Autodesk Fusion 360 part; units mm, degrees
note: some values were not read from the file. Chosen so that the rebuilt part matches the saved one: which face or edge a step refers to. Set by a fixed rule: which sketch regions a step uses.
(part 2 of 4)
sketch "Front projection" plane through (0, 0, 0) normal (0, 0, 1) x (1, 0, 0) in component "Front"
  arc A0 (5.175, 6.81) -> (5.175, 8.2242) centre (4.4679, 7.5171) ccw
  line L0 (5.175, 6.81) -> (5.175, 5.175)
  line L1 (5.175, 58.825) -> (5.175, 57.19)
  arc A1 (5.175, 55.7758) -> (5.175, 57.19) centre (4.4679, 56.4829) ccw
  line L2 (5.175, 55.7758) -> (5.175, 48.2242)
  arc A2 (3.5613, 47.095) -> (5.175, 48.2242) centre (4.4679, 47.5171) ccw
  line L3 (3.5613, 47.095) -> (2, 47.095)
  line L4 (2, 36.905) -> (3.5613, 36.905)
  arc A3 (5.175, 35.7758) -> (3.5613, 36.905) centre (4.4679, 36.4829) ccw
  line L5 (5.175, 35.7758) -> (5.175, 28.2242)
  arc A4 (3.5613, 27.095) -> (5.175, 28.2242) centre (4.4679, 27.5171) ccw
  line L6 (3.5613, 27.095) -> (2, 27.095)
  line L7 (2, 16.905) -> (3.5613, 16.905)
  arc A5 (5.175, 15.7758) -> (3.5613, 16.905) centre (4.4679, 16.4829) ccw
  line L8 (5.175, 15.7758) -> (5.175, 8.2242)
  line L9 (15.7758, 58.825) -> (5.175, 58.825)
  line L10 (2, 16.905) -> (2, 27.095)
  arc A6 (238.825, 8.2242) -> (238.825, 6.81) centre (239.5321, 7.5171) ccw
  line L11 (216.905, 62) -> (216.905, 60.4387)
  arc A7 (215.7758, 58.825) -> (216.905, 60.4387) centre (216.4829, 59.5321) ccw
  line L12 (215.7758, 58.825) -> (208.2242, 58.825)
  arc A8 (207.095, 60.4387) -> (208.2242, 58.825) centre (207.5171, 59.5321) ccw
  line L13 (207.095, 60.4387) -> (207.095, 62)
  line L14 (196.905, 62) -> (196.905, 60.4387)
  arc A9 (195.7758, 58.825) -> (196.905, 60.4387) centre (196.4829, 59.5321) ccw
  line L15 (195.7758, 58.825) -> (188.2242, 58.825)
  arc A10 (187.095, 60.4387) -> (188.2242, 58.825) centre (187.5171, 59.5321) ccw
  line L16 (187.095, 60.4387) -> (187.095, 62)
  line L17 (176.905, 62) -> (176.905, 60.4387)
  arc A11 (175.7758, 58.825) -> (176.905, 60.4387) centre (176.4829, 59.5321) ccw
  line L18 (175.7758, 58.825) -> (168.2242, 58.825)
  arc A12 (167.095, 60.4387) -> (168.2242, 58.825) centre (167.5171, 59.5321) ccw
  line L19 (167.095, 60.4387) -> (167.095, 62)
  line L20 (156.905, 62) -> (156.905, 60.4387)
  arc A13 (155.7758, 58.825) -> (156.905, 60.4387) centre (156.4829, 59.5321) ccw
  line L21 (155.7758, 58.825) -> (148.2242, 58.825)
  arc A14 (147.095, 60.4387) -> (148.2242, 58.825) centre (147.5171, 59.5321) ccw
  line L22 (147.095, 60.4387) -> (147.095, 62)
  line L23 (136.905, 62) -> (136.905, 60.4387)
  arc A15 (135.7758, 58.825) -> (136.905, 60.4387) centre (136.4829, 59.5321) ccw
  line L24 (135.7758, 58.825) -> (128.2242, 58.825)
  arc A16 (127.095, 60.4387) -> (128.2242, 58.825) centre (127.5171, 59.5321) ccw
  line L25 (127.095, 60.4387) -> (127.095, 62)
  line L26 (116.905, 62) -> (116.905, 60.4387)
  arc A17 (115.7758, 58.825) -> (116.905, 60.4387) centre (116.4829, 59.5321) ccw
  line L27 (115.7758, 58.825) -> (108.2242, 58.825)
  arc A18 (107.095, 60.4387) -> (108.2242, 58.825) centre (107.5171, 59.5321) ccw
  line L28 (107.095, 60.4387) -> (107.095, 62)
  line L29 (96.905, 62) -> (96.905, 60.4387)
  arc A19 (95.7758, 58.825) -> (96.905, 60.4387) centre (96.4829, 59.5321) ccw
  line L30 (95.7758, 58.825) -> (88.2242, 58.825)
  arc A20 (87.095, 60.4387) -> (88.2242, 58.825) centre (87.5171, 59.5321) ccw
  line L31 (87.095, 60.4387) -> (87.095, 62)
  line L32 (76.905, 62) -> (76.905, 60.4387)
  arc A21 (75.7758, 58.825) -> (76.905, 60.4387) centre (76.4829, 59.5321) ccw
  line L33 (75.7758, 58.825) -> (68.2242, 58.825)
  arc A22 (67.095, 60.4387) -> (68.2242, 58.825) centre (67.5171, 59.5321) ccw
  line L34 (67.095, 60.4387) -> (67.095, 62)
  line L35 (56.905, 62) -> (56.905, 60.4387)
  arc A23 (55.7758, 58.825) -> (56.905, 60.4387) centre (56.4829, 59.5321) ccw
  line L36 (55.7758, 58.825) -> (48.2242, 58.825)
  arc A24 (47.095, 60.4387) -> (48.2242, 58.825) centre (47.5171, 59.5321) ccw
  line L37 (47.095, 60.4387) -> (47.095, 62)
  line L38 (238.825, 58.825) -> (228.2242, 58.825)
  arc A25 (227.095, 60.4387) -> (228.2242, 58.825) centre (227.5171, 59.5321) ccw
  line L39 (227.095, 60.4387) -> (227.095, 62)
  line L40 (36.905, 62) -> (36.905, 60.4387)
  arc A26 (35.7758, 58.825) -> (36.905, 60.4387) centre (36.4829, 59.5321) ccw
  line L41 (35.7758, 58.825) -> (28.2242, 58.825)
  arc A27 (27.095, 60.4387) -> (28.2242, 58.825) centre (27.5171, 59.5321) ccw
  line L42 (27.095, 60.4387) -> (27.095, 62)
  line L43 (16.905, 62) -> (16.905, 60.4387)
  arc A28 (15.7758, 58.825) -> (16.905, 60.4387) centre (16.4829, 59.5321) ccw
  line L44 (238.825, 5.175) -> (238.825, 6.81)
  line L45 (238.825, 58.825) -> (238.825, 57.19)
  line L46 (16.905, 62) -> (27.095, 62)
  line L47 (36.905, 62) -> (47.095, 62)
  line L48 (56.905, 62) -> (67.095, 62)
  line L49 (76.905, 62) -> (87.095, 62)
  line L50 (96.905, 62) -> (107.095, 62)
  line L51 (116.905, 62) -> (127.095, 62)
  line L52 (136.905, 62) -> (147.095, 62)
  line L53 (156.905, 62) -> (167.095, 62)
  line L54 (176.905, 62) -> (187.095, 62)
  line L55 (196.905, 62) -> (207.095, 62)
  line L56 (216.905, 62) -> (227.095, 62)
  arc A29 (238.825, 57.19) -> (238.825, 55.7758) centre (239.5321, 56.4829) ccw
  line L57 (238.825, 55.7758) -> (238.825, 48.2242)
  arc A30 (238.825, 48.2242) -> (240.4387, 47.095) centre (239.5321, 47.5171) ccw
  line L58 (240.4387, 47.095) -> (242, 47.095)
  line L59 (242, 47.095) -> (242, 36.905)
  line L60 (240.4387, 36.905) -> (242, 36.905)
  arc A31 (240.4387, 36.905) -> (238.825, 35.7758) centre (239.5321, 36.4829) ccw
  line L61 (238.825, 28.2242) -> (238.825, 35.7758)
  arc A32 (238.825, 28.2242) -> (240.4387, 27.095) centre (239.5321, 27.5171) ccw
  line L62 (242, 27.095) -> (240.4387, 27.095)
  line L63 (242, 27.095) -> (242, 16.905)
  line L64 (240.4387, 16.905) -> (242, 16.905)
  arc A33 (240.4387, 16.905) -> (238.825, 15.7758) centre (239.5321, 16.4829) ccw
  line L65 (238.825, 8.2242) -> (238.825, 15.7758)
  line L66 (238.825, 5.175) -> (228.2242, 5.175)
  arc A34 (228.2242, 5.175) -> (227.095, 3.5613) centre (227.5171, 4.4679) ccw
  line L67 (227.095, 3.5613) -> (227.095, 2)
  line L68 (227.095, 2) -> (216.905, 2)
  line L69 (216.905, 3.5613) -> (216.905, 2)
  arc A35 (216.905, 3.5613) -> (215.7758, 5.175) centre (216.4829, 4.4679) ccw
  line L70 (208.2242, 5.175) -> (215.7758, 5.175)
  arc A36 (208.2242, 5.175) -> (207.095, 3.5613) centre (207.5171, 4.4679) ccw
  line L71 (207.095, 2) -> (207.095, 3.5613)
  line L72 (207.095, 2) -> (196.905, 2)
  line L73 (196.905, 3.5613) -> (196.905, 2)
  arc A37 (196.905, 3.5613) -> (195.7758, 5.175) centre (196.4829, 4.4679) ccw
  line L74 (188.2242, 5.175) -> (195.7758, 5.175)
  arc A38 (188.2242, 5.175) -> (187.095, 3.5613) centre (187.5171, 4.4679) ccw
  line L75 (187.095, 2) -> (187.095, 3.5613)
  line L76 (187.095, 2) -> (176.905, 2)
  line L77 (176.905, 3.5613) -> (176.905, 2)
  arc A39 (176.905, 3.5613) -> (175.7758, 5.175) centre (176.4829, 4.4679) ccw
  line L78 (168.2242, 5.175) -> (175.7758, 5.175)
  arc A40 (168.2242, 5.175) -> (167.095, 3.5613) centre (167.5171, 4.4679) ccw
  line L79 (167.095, 2) -> (167.095, 3.5613)
  line L80 (167.095, 2) -> (156.905, 2)
  line L81 (156.905, 3.5613) -> (156.905, 2)
  arc A41 (156.905, 3.5613) -> (155.7758, 5.175) centre (156.4829, 4.4679) ccw
  line L82 (148.2242, 5.175) -> (155.7758, 5.175)
  arc A42 (148.2242, 5.175) -> (147.095, 3.5613) centre (147.5171, 4.4679) ccw
  line L83 (147.095, 2) -> (147.095, 3.5613)
  line L84 (147.095, 2) -> (136.905, 2)
  line L85 (136.905, 3.5613) -> (136.905, 2)
  arc A43 (136.905, 3.5613) -> (135.7758, 5.175) centre (136.4829, 4.4679) ccw
  line L86 (128.2242, 5.175) -> (135.7758, 5.175)
  arc A44 (128.2242, 5.175) -> (127.095, 3.5613) centre (127.5171, 4.4679) ccw
  line L87 (127.095, 2) -> (127.095, 3.5613)
  line L88 (127.095, 2) -> (116.905, 2)
  line L89 (116.905, 3.5613) -> (116.905, 2)
  arc A45 (116.905, 3.5613) -> (115.7758, 5.175) centre (116.4829, 4.4679) ccw
  line L90 (108.2242, 5.175) -> (115.7758, 5.175)
  arc A46 (108.2242, 5.175) -> (107.095, 3.5613) centre (107.5171, 4.4679) ccw
  line L91 (107.095, 2) -> (107.095, 3.5613)
  line L92 (107.095, 2) -> (96.905, 2)
  line L93 (96.905, 3.5613) -> (96.905, 2)
  arc A47 (96.905, 3.5613) -> (95.7758, 5.175) centre (96.4829, 4.4679) ccw
  line L94 (88.2242, 5.175) -> (95.7758, 5.175)
  arc A48 (88.2242, 5.175) -> (87.095, 3.5613) centre (87.5171, 4.4679) ccw
  line L95 (87.095, 2) -> (87.095, 3.5613)
  line L96 (87.095, 2) -> (76.905, 2)
  line L97 (76.905, 3.5613) -> (76.905, 2)
  arc A49 (76.905, 3.5613) -> (75.7758, 5.175) centre (76.4829, 4.4679) ccw
  line L98 (68.2242, 5.175) -> (75.7758, 5.175)
  arc A50 (68.2242, 5.175) -> (67.095, 3.5613) centre (67.5171, 4.4679) ccw
  line L99 (67.095, 2) -> (67.095, 3.5613)
  line L100 (67.095, 2) -> (56.905, 2)
  line L101 (56.905, 3.5613) -> (56.905, 2)
  arc A51 (56.905, 3.5613) -> (55.7758, 5.175) centre (56.4829, 4.4679) ccw
  line L102 (48.2242, 5.175) -> (55.7758, 5.175)
  arc A52 (48.2242, 5.175) -> (47.095, 3.5613) centre (47.5171, 4.4679) ccw
  line L103 (47.095, 2) -> (47.095, 3.5613)
  line L104 (47.095, 2) -> (36.905, 2)
  line L105 (36.905, 3.5613) -> (36.905, 2)
  arc A53 (36.905, 3.5613) -> (35.7758, 5.175) centre (36.4829, 4.4679) ccw
  line L106 (28.2242, 5.175) -> (35.7758, 5.175)
  arc A54 (28.2242, 5.175) -> (27.095, 3.5613) centre (27.5171, 4.4679) ccw
  line L107 (27.095, 2) -> (27.095, 3.5613)
  line L108 (27.095, 2) -> (16.905, 2)
  line L109 (16.905, 3.5613) -> (16.905, 2)
  arc A55 (16.905, 3.5613) -> (15.7758, 5.175) centre (16.4829, 4.4679) ccw
  line L110 (5.175, 5.175) -> (15.7758, 5.175)
  line L111 (2, 36.905) -> (2, 47.095)
sketch "Right Projection" plane through (0, 0, 0) normal (0, 0, 1) x (1, 0, 0) in component "Right"
  line L0 (-300.4387, 26.095) -> (-302, 26.095)
  line L1 (-302, 35.905) -> (-300.4387, 35.905)
  arc A0 (-298.825, 34.7758) -> (-300.4387, 35.905) centre (-299.5321, 35.4829) ccw
  line L2 (-298.825, 34.7758) -> (-298.825, 27.2242)
  arc A1 (-300.4387, 26.095) -> (-298.825, 27.2242) centre (-299.5321, 26.5171) ccw
  line L3 (-302, 55.905) -> (-300.4387, 55.905)
  line L4 (-300.4387, 46.095) -> (-302, 46.095)
  arc A2 (-300.4387, 46.095) -> (-298.825, 47.2242) centre (-299.5321, 46.5171) ccw
  line L5 (-298.825, 54.7758) -> (-298.825, 47.2242)
  arc A3 (-298.825, 54.7758) -> (-300.4387, 55.905) centre (-299.5321, 55.4829) ccw
  line L6 (-302, 75.905) -> (-300.4387, 75.905)
  line L7 (-300.4387, 66.095) -> (-302, 66.095)
  arc A4 (-300.4387, 66.095) -> (-298.825, 67.2242) centre (-299.5321, 66.5171) ccw
  line L8 (-298.825, 74.7758) -> (-298.825, 67.2242)
  arc A5 (-298.825, 74.7758) -> (-300.4387, 75.905) centre (-299.5321, 75.4829) ccw
  line L9 (-302, 95.905) -> (-300.4387, 95.905)
  line L10 (-300.4387, 86.095) -> (-302, 86.095)
  arc A6 (-300.4387, 86.095) -> (-298.825, 87.2242) centre (-299.5321, 86.5171) ccw
  line L11 (-298.825, 94.7758) -> (-298.825, 87.2242)
  arc A7 (-298.825, 94.7758) -> (-300.4387, 95.905) centre (-299.5321, 95.4829) ccw
  line L12 (-302, 115.905) -> (-300.4387, 115.905)
  line L13 (-300.4387, 106.095) -> (-302, 106.095)
  arc A8 (-300.4387, 106.095) -> (-298.825, 107.2242) centre (-299.5321, 106.5171) ccw
  line L14 (-298.825, 114.7758) -> (-298.825, 107.2242)
  arc A9 (-298.825, 114.7758) -> (-300.4387, 115.905) centre (-299.5321, 115.4829) ccw
  line L15 (-302, 135.905) -> (-300.4387, 135.905)
  line L16 (-300.4387, 126.095) -> (-302, 126.095)
  arc A10 (-300.4387, 126.095) -> (-298.825, 127.2242) centre (-299.5321, 126.5171) ccw
  line L17 (-298.825, 134.7758) -> (-298.825, 127.2242)
  arc A11 (-298.825, 134.7758) -> (-300.4387, 135.905) centre (-299.5321, 135.4829) ccw
  line L18 (-302, 155.905) -> (-300.4387, 155.905)
  line L19 (-300.4387, 166.095) -> (-302, 166.095)
  arc A12 (-300.4387, 166.095) -> (-298.825, 167.2242) centre (-299.5321, 166.5171) ccw
  line L20 (-298.825, 182) -> (-298.825, 167.2242)
  line L21 (-298.825, 14.7758) -> (-298.825, 0)
  arc A13 (-298.825, 14.7758) -> (-300.4387, 15.905) centre (-299.5321, 15.4829) ccw
  line L22 (-302, 15.905) -> (-300.4387, 15.905)
  line L23 (-300.4387, 146.095) -> (-302, 146.095)
  arc A14 (-300.4387, 146.095) -> (-298.825, 147.2242) centre (-299.5321, 146.5171) ccw
  line L24 (-298.825, 154.7758) -> (-298.825, 147.2242)
  arc A15 (-298.825, 154.7758) -> (-300.4387, 155.905) centre (-299.5321, 155.4829) ccw
  line L25 (-298.825, 0) -> (-286.905, 0)
  line L26 (-302, 26.095) -> (-302, 15.905)
  line L27 (-302, 46.095) -> (-302, 35.905)
  line L28 (-302, 66.095) -> (-302, 55.905)
  line L29 (-302, 86.095) -> (-302, 75.905)
  line L30 (-302, 106.095) -> (-302, 95.905)
  line L31 (-302, 126.095) -> (-302, 115.905)
  line L32 (-302, 146.095) -> (-302, 135.905)
  line L33 (-302, 166.095) -> (-302, 155.905)
  line L34 (-286.905, 182) -> (-298.825, 182)
  line L35 (-286.905, 182) -> (-286.905, 180.4387)
  arc A16 (-286.905, 180.4387) -> (-285.7758, 178.825) centre (-286.4829, 179.5321) ccw
  line L36 (-285.7758, 178.825) -> (-278.2242, 178.825)
  arc A17 (-278.2242, 178.825) -> (-277.095, 180.4387) centre (-277.5171, 179.5321) ccw
  line L37 (-277.095, 180.4387) -> (-277.095, 182)
  line L38 (-266.905, 182) -> (-277.095, 182)
  line L39 (-266.905, 182) -> (-266.905, 180.4387)
  arc A18 (-266.905, 180.4387) -> (-265.7758, 178.825) centre (-266.4829, 179.5321) ccw
  line L40 (-265.7758, 178.825) -> (-258.2242, 178.825)
  arc A19 (-258.2242, 178.825) -> (-257.095, 180.4387) centre (-257.5171, 179.5321) ccw
  line L41 (-257.095, 180.4387) -> (-257.095, 182)
  line L42 (-245.175, 182) -> (-257.095, 182)
  line L43 (-245.175, 182) -> (-245.175, 167.2242)
  arc A20 (-245.175, 167.2242) -> (-243.5613, 166.095) centre (-244.4679, 166.5171) ccw
  line L44 (-243.5613, 166.095) -> (-242, 166.095)
  line L45 (-242, 155.905) -> (-242, 166.095)
  line L46 (-242, 155.905) -> (-243.5613, 155.905)
  arc A21 (-243.5613, 155.905) -> (-245.175, 154.7758) centre (-244.4679, 155.4829) ccw
  line L47 (-245.175, 154.7758) -> (-245.175, 147.2242)
  arc A22 (-245.175, 147.2242) -> (-243.5613, 146.095) centre (-244.4679, 146.5171) ccw
  line L48 (-243.5613, 146.095) -> (-242, 146.095)
  line L49 (-242, 135.905) -> (-242, 146.095)
  line L50 (-242, 135.905) -> (-243.5613, 135.905)
  arc A23 (-243.5613, 135.905) -> (-245.175, 134.7758) centre (-244.4679, 135.4829) ccw
  line L51 (-245.175, 134.7758) -> (-245.175, 127.2242)
  arc A24 (-245.175, 127.2242) -> (-243.5613, 126.095) centre (-244.4679, 126.5171) ccw
  line L52 (-243.5613, 126.095) -> (-242, 126.095)
  line L53 (-242, 115.905) -> (-242, 126.095)
  line L54 (-242, 115.905) -> (-243.5613, 115.905)
  arc A25 (-243.5613, 115.905) -> (-245.175, 114.7758) centre (-244.4679, 115.4829) ccw
  line L55 (-245.175, 114.7758) -> (-245.175, 107.2242)
  arc A26 (-245.175, 107.2242) -> (-243.5613, 106.095) centre (-244.4679, 106.5171) ccw
  line L56 (-243.5613, 106.095) -> (-242, 106.095)
  line L57 (-242, 95.905) -> (-242, 106.095)
  line L58 (-242, 95.905) -> (-243.5613, 95.905)
  arc A27 (-243.5613, 95.905) -> (-245.175, 94.7758) centre (-244.4679, 95.4829) ccw
  line L59 (-245.175, 94.7758) -> (-245.175, 87.2242)
  arc A28 (-245.175, 87.2242) -> (-243.5613, 86.095) centre (-244.4679, 86.5171) ccw
  line L60 (-243.5613, 86.095) -> (-242, 86.095)
  line L61 (-242, 75.905) -> (-242, 86.095)
  line L62 (-242, 75.905) -> (-243.5613, 75.905)
  arc A29 (-243.5613, 75.905) -> (-245.175, 74.7758) centre (-244.4679, 75.4829) ccw
  line L63 (-245.175, 74.7758) -> (-245.175, 67.2242)
  arc A30 (-245.175, 67.2242) -> (-243.5613, 66.095) centre (-244.4679, 66.5171) ccw
  line L64 (-243.5613, 66.095) -> (-242, 66.095)
  line L65 (-242, 55.905) -> (-242, 66.095)
  line L66 (-242, 55.905) -> (-243.5613, 55.905)
  arc A31 (-243.5613, 55.905) -> (-245.175, 54.7758) centre (-244.4679, 55.4829) ccw
  line L67 (-245.175, 54.7758) -> (-245.175, 47.2242)
  arc A32 (-245.175, 47.2242) -> (-243.5613, 46.095) centre (-244.4679, 46.5171) ccw
  line L68 (-243.5613, 46.095) -> (-242, 46.095)
  line L69 (-242, 35.905) -> (-242, 46.095)
  line L70 (-243.5613, 35.905) -> (-242, 35.905)
  arc A33 (-243.5613, 35.905) -> (-245.175, 34.7758) centre (-244.4679, 35.4829) ccw
  line L71 (-245.175, 27.2242) -> (-245.175, 34.7758)
  arc A34 (-245.175, 27.2242) -> (-243.5613, 26.095) centre (-244.4679, 26.5171) ccw
  line L72 (-242, 26.095) -> (-243.5613, 26.095)
  line L73 (-242, 15.905) -> (-242, 26.095)
  line L74 (-243.5613, 15.905) -> (-242, 15.905)
  arc A35 (-243.5613, 15.905) -> (-245.175, 14.7758) centre (-244.4679, 15.4829) ccw
  line L75 (-245.175, 0) -> (-245.175, 14.7758)
  line L76 (-257.095, 0) -> (-245.175, 0)
  line L77 (-257.095, 1.5613) -> (-257.095, 0)
  arc A36 (-257.095, 1.5613) -> (-258.2242, 3.175) centre (-257.5171, 2.4679) ccw
  line L78 (-265.7758, 3.175) -> (-258.2242, 3.175)
  arc A37 (-265.7758, 3.175) -> (-266.905, 1.5613) centre (-266.4829, 2.4679) ccw
  line L79 (-266.905, 0) -> (-266.905, 1.5613)
  line L80 (-277.095, 0) -> (-266.905, 0)
  line L81 (-277.095, 1.5613) -> (-277.095, 0)
  arc A38 (-277.095, 1.5613) -> (-278.2242, 3.175) centre (-277.5171, 2.4679) ccw
  line L82 (-285.7758, 3.175) -> (-278.2242, 3.175)
  arc A39 (-285.7758, 3.175) -> (-286.905, 1.5613) centre (-286.4829, 2.4679) ccw
  line L83 (-286.905, 0) -> (-286.905, 1.5613)
sketch "Left Projection" plane through (0, 0, 0) normal (0, 0, 1) x (1, 0, 0) in component "Left"
  line L0 (-300.4387, -28.095) -> (-302, -28.095)
  line L1 (-302, -37.905) -> (-300.4387, -37.905)
  arc A0 (-300.4387, -37.905) -> (-298.825, -36.7758) centre (-299.5321, -37.4829) ccw
  line L2 (-298.825, -36.7758) -> (-298.825, -29.2242)
  arc A1 (-298.825, -29.2242) -> (-300.4387, -28.095) centre (-299.5321, -28.5171) ccw
  line L3 (-302, -57.905) -> (-300.4387, -57.905)
  line L4 (-300.4387, -48.095) -> (-302, -48.095)
  arc A2 (-298.825, -49.2242) -> (-300.4387, -48.095) centre (-299.5321, -48.5171) ccw
  line L5 (-298.825, -56.7758) -> (-298.825, -49.2242)
  arc A3 (-300.4387, -57.905) -> (-298.825, -56.7758) centre (-299.5321, -57.4829) ccw
  line L6 (-302, -77.905) -> (-300.4387, -77.905)
  line L7 (-300.4387, -68.095) -> (-302, -68.095)
  arc A4 (-298.825, -69.2242) -> (-300.4387, -68.095) centre (-299.5321, -68.5171) ccw
  line L8 (-298.825, -76.7758) -> (-298.825, -69.2242)
  arc A5 (-300.4387, -77.905) -> (-298.825, -76.7758) centre (-299.5321, -77.4829) ccw
  line L9 (-302, -97.905) -> (-300.4387, -97.905)
  line L10 (-300.4387, -88.095) -> (-302, -88.095)
  arc A6 (-298.825, -89.2242) -> (-300.4387, -88.095) centre (-299.5321, -88.5171) ccw
  line L11 (-298.825, -96.7758) -> (-298.825, -89.2242)
  arc A7 (-300.4387, -97.905) -> (-298.825, -96.7758) centre (-299.5321, -97.4829) ccw
  line L12 (-302, -117.905) -> (-300.4387, -117.905)
  line L13 (-300.4387, -108.095) -> (-302, -108.095)
  arc A8 (-298.825, -109.2242) -> (-300.4387, -108.095) centre (-299.5321, -108.5171) ccw
  line L14 (-298.825, -116.7758) -> (-298.825, -109.2242)
  arc A9 (-300.4387, -117.905) -> (-298.825, -116.7758) centre (-299.5321, -117.4829) ccw
  line L15 (-302, -137.905) -> (-300.4387, -137.905)
  line L16 (-300.4387, -128.095) -> (-302, -128.095)
  arc A10 (-298.825, -129.2242) -> (-300.4387, -128.095) centre (-299.5321, -128.5171) ccw
  line L17 (-298.825, -136.7758) -> (-298.825, -129.2242)
  arc A11 (-300.4387, -137.905) -> (-298.825, -136.7758) centre (-299.5321, -137.4829) ccw
  line L18 (-302, -157.905) -> (-300.4387, -157.905)
  line L19 (-300.4387, -168.095) -> (-302, -168.095)
  arc A12 (-298.825, -169.2242) -> (-300.4387, -168.095) centre (-299.5321, -168.5171) ccw
  line L20 (-298.825, -184) -> (-298.825, -169.2242)
  line L21 (-298.825, -16.7758) -> (-298.825, -2)
  arc A13 (-300.4387, -17.905) -> (-298.825, -16.7758) centre (-299.5321, -17.4829) ccw
  line L22 (-302, -17.905) -> (-300.4387, -17.905)
  line L23 (-300.4387, -148.095) -> (-302, -148.095)
  arc A14 (-298.825, -149.2242) -> (-300.4387, -148.095) centre (-299.5321, -148.5171) ccw
  line L24 (-298.825, -156.7758) -> (-298.825, -149.2242)
  arc A15 (-300.4387, -157.905) -> (-298.825, -156.7758) centre (-299.5321, -157.4829) ccw
  line L25 (-298.825, -2) -> (-286.905, -2)
  line L26 (-286.905, -2) -> (-286.905, -3.5613)
  arc A16 (-286.905, -3.5613) -> (-285.7758, -5.175) centre (-286.4829, -4.4679) ccw
  line L27 (-285.7758, -5.175) -> (-278.2242, -5.175)
  arc A17 (-278.2242, -5.175) -> (-277.095, -3.5613) centre (-277.5171, -4.4679) ccw
  line L28 (-277.095, -3.5613) -> (-277.095, -2)
  line L29 (-277.095, -2) -> (-266.905, -2)
  line L30 (-266.905, -2) -> (-266.905, -3.5613)
  arc A18 (-266.905, -3.5613) -> (-265.7758, -5.175) centre (-266.4829, -4.4679) ccw
  line L31 (-265.7758, -5.175) -> (-258.2242, -5.175)
  arc A19 (-258.2242, -5.175) -> (-257.095, -3.5613) centre (-257.5171, -4.4679) ccw
  line L32 (-257.095, -3.5613) -> (-257.095, -2)
  line L33 (-257.095, -2) -> (-245.175, -2)
  line L34 (-245.175, -2) -> (-245.175, -16.7758)
  arc A20 (-245.175, -16.7758) -> (-243.5613, -17.905) centre (-244.4679, -17.4829) ccw
  line L35 (-243.5613, -17.905) -> (-242, -17.905)
  line L36 (-242, -17.905) -> (-242, -28.095)
  line L37 (-242, -28.095) -> (-243.5613, -28.095)
  arc A21 (-243.5613, -28.095) -> (-245.175, -29.2242) centre (-244.4679, -28.5171) ccw
  line L38 (-245.175, -29.2242) -> (-245.175, -36.7758)
  arc A22 (-245.175, -36.7758) -> (-243.5613, -37.905) centre (-244.4679, -37.4829) ccw
  line L39 (-243.5613, -37.905) -> (-242, -37.905)
  line L40 (-242, -37.905) -> (-242, -48.095)
  line L41 (-243.5613, -48.095) -> (-242, -48.095)
  arc A23 (-243.5613, -48.095) -> (-245.175, -49.2242) centre (-244.4679, -48.5171) ccw
  line L42 (-245.175, -56.7758) -> (-245.175, -49.2242)
  arc A24 (-245.175, -56.7758) -> (-243.5613, -57.905) centre (-244.4679, -57.4829) ccw
  line L43 (-242, -57.905) -> (-243.5613, -57.905)
  line L44 (-242, -57.905) -> (-242, -68.095)
  line L45 (-243.5613, -68.095) -> (-242, -68.095)
  arc A25 (-243.5613, -68.095) -> (-245.175, -69.2242) centre (-244.4679, -68.5171) ccw
  line L46 (-245.175, -76.7758) -> (-245.175, -69.2242)
  arc A26 (-245.175, -76.7758) -> (-243.5613, -77.905) centre (-244.4679, -77.4829) ccw
  line L47 (-242, -77.905) -> (-243.5613, -77.905)
  line L48 (-242, -77.905) -> (-242, -88.095)
  line L49 (-243.5613, -88.095) -> (-242, -88.095)
  arc A27 (-243.5613, -88.095) -> (-245.175, -89.2242) centre (-244.4679, -88.5171) ccw
  line L50 (-245.175, -96.7758) -> (-245.175, -89.2242)
  arc A28 (-245.175, -96.7758) -> (-243.5613, -97.905) centre (-244.4679, -97.4829) ccw
  line L51 (-242, -97.905) -> (-243.5613, -97.905)
  line L52 (-242, -97.905) -> (-242, -108.095)
  line L53 (-243.5613, -108.095) -> (-242, -108.095)
  arc A29 (-243.5613, -108.095) -> (-245.175, -109.2242) centre (-244.4679, -108.5171) ccw
  line L54 (-245.175, -116.7758) -> (-245.175, -109.2242)
  arc A30 (-245.175, -116.7758) -> (-243.5613, -117.905) centre (-244.4679, -117.4829) ccw
  line L55 (-242, -117.905) -> (-243.5613, -117.905)
  line L56 (-242, -117.905) -> (-242, -128.095)
  line L57 (-243.5613, -128.095) -> (-242, -128.095)
  arc A31 (-243.5613, -128.095) -> (-245.175, -129.2242) centre (-244.4679, -128.5171) ccw
  line L58 (-245.175, -136.7758) -> (-245.175, -129.2242)
  arc A32 (-245.175, -136.7758) -> (-243.5613, -137.905) centre (-244.4679, -137.4829) ccw
  line L59 (-242, -137.905) -> (-243.5613, -137.905)
  line L60 (-242, -137.905) -> (-242, -148.095)
  line L61 (-243.5613, -148.095) -> (-242, -148.095)
  arc A33 (-243.5613, -148.095) -> (-245.175, -149.2242) centre (-244.4679, -148.5171) ccw
  line L62 (-245.175, -156.7758) -> (-245.175, -149.2242)
  arc A34 (-245.175, -156.7758) -> (-243.5613, -157.905) centre (-244.4679, -157.4829) ccw
  line L63 (-242, -157.905) -> (-243.5613, -157.905)
  line L64 (-242, -157.905) -> (-242, -168.095)
  line L65 (-243.5613, -168.095) -> (-242, -168.095)
  arc A35 (-243.5613, -168.095) -> (-245.175, -169.2242) centre (-244.4679, -168.5171) ccw
  line L66 (-245.175, -184) -> (-245.175, -169.2242)
  line L67 (-245.175, -184) -> (-257.095, -184)
  line L68 (-257.095, -182.4387) -> (-257.095, -184)
  arc A36 (-257.095, -182.4387) -> (-258.2242, -180.825) centre (-257.5171, -181.5321) ccw
  line L69 (-265.7758, -180.825) -> (-258.2242, -180.825)
  arc A37 (-265.7758, -180.825) -> (-266.905, -182.4387) centre (-266.4829, -181.5321) ccw
  line L70 (-266.905, -184) -> (-266.905, -182.4387)
  line L71 (-266.905, -184) -> (-277.095, -184)
  line L72 (-277.095, -182.4387) -> (-277.095, -184)
  arc A38 (-277.095, -182.4387) -> (-278.2242, -180.825) centre (-277.5171, -181.5321) ccw
  line L73 (-285.7758, -180.825) -> (-278.2242, -180.825)
  arc A39 (-285.7758, -180.825) -> (-286.905, -182.4387) centre (-286.4829, -181.5321) ccw
  line L74 (-286.905, -184) -> (-286.905, -182.4387)
  line L75 (-286.905, -184) -> (-298.825, -184)
  line L76 (-302, -168.095) -> (-302, -157.905)
  line L77 (-302, -148.095) -> (-302, -137.905)
  line L78 (-302, -128.095) -> (-302, -117.905)
  line L79 (-302, -108.095) -> (-302, -97.905)
  line L80 (-302, -88.095) -> (-302, -77.905)
  line L81 (-302, -68.095) -> (-302, -57.905)
  line L82 (-302, -48.095) -> (-302, -37.905)
  line L83 (-302, -28.095) -> (-302, -17.905)
move_body "Move1" [suppressed] in component "Back"
sketch "Back Projection" plane through (0, 0, 0) normal (0, 0, 1) x (1, 0, 0) in component "Back"
  line L0 (5.175, -60.591) -> (5.175, -62.226)
  line L1 (5.175, -62.226) -> (15.7758, -62.226)
  arc A0 (16.905, -63.8397) -> (15.7758, -62.226) centre (16.4829, -62.9331) ccw
  line L2 (16.905, -63.8397) -> (16.905, -65.401)
  line L3 (16.905, -65.401) -> (27.095, -65.401)
  line L4 (27.095, -65.401) -> (27.095, -63.8397)
  arc A1 (28.2242, -62.226) -> (27.095, -63.8397) centre (27.5171, -62.9331) ccw
  line L5 (28.2242, -62.226) -> (35.7758, -62.226)
  arc A2 (36.905, -63.8397) -> (35.7758, -62.226) centre (36.4829, -62.9331) ccw
  line L6 (36.905, -63.8397) -> (36.905, -65.401)
  line L7 (36.905, -65.401) -> (47.095, -65.401)
  line L8 (47.095, -65.401) -> (47.095, -63.8397)
  arc A3 (48.2242, -62.226) -> (47.095, -63.8397) centre (47.5171, -62.9331) ccw
  line L9 (48.2242, -62.226) -> (55.7758, -62.226)
  arc A4 (56.905, -63.8397) -> (55.7758, -62.226) centre (56.4829, -62.9331) ccw
  line L10 (56.905, -63.8397) -> (56.905, -65.401)
  line L11 (56.905, -65.401) -> (67.095, -65.401)
  line L12 (67.095, -65.401) -> (67.095, -63.8397)
  arc A5 (68.2242, -62.226) -> (67.095, -63.8397) centre (67.5171, -62.9331) ccw
  line L13 (68.2242, -62.226) -> (75.7758, -62.226)
  arc A6 (76.905, -63.8397) -> (75.7758, -62.226) centre (76.4829, -62.9331) ccw
  line L14 (76.905, -63.8397) -> (76.905, -65.401)
  line L15 (76.905, -65.401) -> (87.095, -65.401)
  line L16 (87.095, -65.401) -> (87.095, -63.8397)
  arc A7 (88.2242, -62.226) -> (87.095, -63.8397) centre (87.5171, -62.9331) ccw
  line L17 (88.2242, -62.226) -> (95.7758, -62.226)
  arc A8 (96.905, -63.8397) -> (95.7758, -62.226) centre (96.4829, -62.9331) ccw
  line L18 (96.905, -63.8397) -> (96.905, -65.401)
  line L19 (96.905, -65.401) -> (107.095, -65.401)
  line L20 (107.095, -65.401) -> (107.095, -63.8397)
  arc A9 (108.2242, -62.226) -> (107.095, -63.8397) centre (107.5171, -62.9331) ccw
  line L21 (108.2242, -62.226) -> (115.7758, -62.226)
  arc A10 (116.905, -63.8397) -> (115.7758, -62.226) centre (116.4829, -62.9331) ccw
  line L22 (116.905, -63.8397) -> (116.905, -65.401)
  line L23 (116.905, -65.401) -> (127.095, -65.401)
  line L24 (127.095, -65.401) -> (127.095, -63.8397)
  arc A11 (128.2242, -62.226) -> (127.095, -63.8397) centre (127.5171, -62.9331) ccw
  line L25 (128.2242, -62.226) -> (135.7758, -62.226)
  arc A12 (136.905, -63.8397) -> (135.7758, -62.226) centre (136.4829, -62.9331) ccw
  line L26 (136.905, -63.8397) -> (136.905, -65.401)
  line L27 (136.905, -65.401) -> (147.095, -65.401)
  line L28 (147.095, -65.401) -> (147.095, -63.8397)
  arc A13 (148.2242, -62.226) -> (147.095, -63.8397) centre (147.5171, -62.9331) ccw
  line L29 (148.2242, -62.226) -> (155.7758, -62.226)
  arc A14 (156.905, -63.8397) -> (155.7758, -62.226) centre (156.4829, -62.9331) ccw
  line L30 (156.905, -63.8397) -> (156.905, -65.401)
  line L31 (156.905, -65.401) -> (167.095, -65.401)
  line L32 (167.095, -65.401) -> (167.095, -63.8397)
  arc A15 (168.2242, -62.226) -> (167.095, -63.8397) centre (167.5171, -62.9331) ccw
  line L33 (168.2242, -62.226) -> (175.7758, -62.226)
  arc A16 (176.905, -63.8397) -> (175.7758, -62.226) centre (176.4829, -62.9331) ccw
  line L34 (176.905, -63.8397) -> (176.905, -65.401)
  line L35 (176.905, -65.401) -> (187.095, -65.401)
  line L36 (187.095, -65.401) -> (187.095, -63.8397)
  arc A17 (188.2242, -62.226) -> (187.095, -63.8397) centre (187.5171, -62.9331) ccw
  line L37 (188.2242, -62.226) -> (195.7758, -62.226)
  arc A18 (196.905, -63.8397) -> (195.7758, -62.226) centre (196.4829, -62.9331) ccw
  line L38 (196.905, -63.8397) -> (196.905, -65.401)
  line L39 (196.905, -65.401) -> (207.095, -65.401)
  line L40 (207.095, -65.401) -> (207.095, -63.8397)
  arc A19 (208.2242, -62.226) -> (207.095, -63.8397) centre (207.5171, -62.9331) ccw
  line L41 (208.2242, -62.226) -> (215.7758, -62.226)
  arc A20 (216.905, -63.8397) -> (215.7758, -62.226) centre (216.4829, -62.9331) ccw
  line L42 (216.905, -63.8397) -> (216.905, -65.401)
  line L43 (216.905, -65.401) -> (227.095, -65.401)
  line L44 (227.095, -65.401) -> (227.095, -63.8397)
  arc A21 (228.2242, -62.226) -> (227.095, -63.8397) centre (227.5171, -62.9331) ccw
  line L45 (228.2242, -62.226) -> (238.825, -62.226)
  line L46 (238.825, -62.226) -> (238.825, -60.591)
  arc A22 (238.825, -59.1768) -> (238.825, -60.591) centre (239.5321, -59.8839) ccw
  line L47 (238.825, -59.1768) -> (238.825, -51.6252)
  arc A23 (240.4387, -50.496) -> (238.825, -51.6252) centre (239.5321, -50.9181) ccw
  line L48 (240.4387, -50.496) -> (242, -50.496)
  line L49 (242, -50.496) -> (242, -40.306)
  line L50 (242, -40.306) -> (240.4387, -40.306)
  arc A24 (238.825, -39.1768) -> (240.4387, -40.306) centre (239.5321, -39.8839) ccw
  line L51 (238.825, -39.1768) -> (238.825, -31.6252)
  arc A25 (240.4387, -30.496) -> (238.825, -31.6252) centre (239.5321, -30.9181) ccw
  line L52 (240.4387, -30.496) -> (242, -30.496)
  line L53 (242, -30.496) -> (242, -20.306)
  line L54 (242, -20.306) -> (240.4387, -20.306)
  arc A26 (238.825, -19.1768) -> (240.4387, -20.306) centre (239.5321, -19.8839) ccw
  line L55 (238.825, -19.1768) -> (238.825, -11.6252)
  arc A27 (238.825, -10.211) -> (238.825, -11.6252) centre (239.5321, -10.9181) ccw
  line L56 (238.825, -10.211) -> (238.825, -8.576)
  line L57 (238.825, -8.576) -> (228.2242, -8.576)
  arc A28 (227.095, -6.9623) -> (228.2242, -8.576) centre (227.5171, -7.8689) ccw
  line L58 (227.095, -6.9623) -> (227.095, -5.401)
  line L59 (227.095, -5.401) -> (216.905, -5.401)
  line L60 (216.905, -5.401) -> (216.905, -6.9623)
  arc A29 (215.7758, -8.576) -> (216.905, -6.9623) centre (216.4829, -7.8689) ccw
  line L61 (215.7758, -8.576) -> (208.2242, -8.576)
  arc A30 (207.095, -6.9623) -> (208.2242, -8.576) centre (207.5171, -7.8689) ccw
  line L62 (207.095, -6.9623) -> (207.095, -5.401)
  line L63 (207.095, -5.401) -> (196.905, -5.401)
  line L64 (196.905, -5.401) -> (196.905, -6.9623)
  arc A31 (195.7758, -8.576) -> (196.905, -6.9623) centre (196.4829, -7.8689) ccw
  line L65 (195.7758, -8.576) -> (188.2242, -8.576)
  arc A32 (187.095, -6.9623) -> (188.2242, -8.576) centre (187.5171, -7.8689) ccw
  line L66 (187.095, -6.9623) -> (187.095, -5.401)
  line L67 (187.095, -5.401) -> (176.905, -5.401)
  line L68 (176.905, -5.401) -> (176.905, -6.9623)
  arc A33 (175.7758, -8.576) -> (176.905, -6.9623) centre (176.4829, -7.8689) ccw
  line L69 (175.7758, -8.576) -> (168.2242, -8.576)
  arc A34 (167.095, -6.9623) -> (168.2242, -8.576) centre (167.5171, -7.8689) ccw
  line L70 (167.095, -6.9623) -> (167.095, -5.401)
  line L71 (167.095, -5.401) -> (156.905, -5.401)
  line L72 (156.905, -5.401) -> (156.905, -6.9623)
  arc A35 (155.7758, -8.576) -> (156.905, -6.9623) centre (156.4829, -7.8689) ccw
  line L73 (155.7758, -8.576) -> (148.2242, -8.576)
  arc A36 (147.095, -6.9623) -> (148.2242, -8.576) centre (147.5171, -7.8689) ccw
  line L74 (147.095, -6.9623) -> (147.095, -5.401)
  line L75 (147.095, -5.401) -> (136.905, -5.401)
  line L76 (136.905, -5.401) -> (136.905, -6.9623)
  arc A37 (135.7758, -8.576) -> (136.905, -6.9623) centre (136.4829, -7.8689) ccw
  line L77 (135.7758, -8.576) -> (128.2242, -8.576)
  arc A38 (127.095, -6.9623) -> (128.2242, -8.576) centre (127.5171, -7.8689) ccw
  line L78 (127.095, -6.9623) -> (127.095, -5.401)
  line L79 (127.095, -5.401) -> (116.905, -5.401)
  line L80 (116.905, -5.401) -> (116.905, -6.9623)
  arc A39 (115.7758, -8.576) -> (116.905, -6.9623) centre (116.4829, -7.8689) ccw
  line L81 (115.7758, -8.576) -> (108.2242, -8.576)
  arc A40 (107.095, -6.9623) -> (108.2242, -8.576) centre (107.5171, -7.8689) ccw
  line L82 (107.095, -6.9623) -> (107.095, -5.401)
  line L83 (107.095, -5.401) -> (96.905, -5.401)
  line L84 (96.905, -5.401) -> (96.905, -6.9623)
  arc A41 (95.7758, -8.576) -> (96.905, -6.9623) centre (96.4829, -7.8689) ccw
  line L85 (95.7758, -8.576) -> (88.2242, -8.576)
  arc A42 (87.095, -6.9623) -> (88.2242, -8.576) centre (87.5171, -7.8689) ccw
  line L86 (87.095, -6.9623) -> (87.095, -5.401)
  line L87 (87.095, -5.401) -> (76.905, -5.401)
  line L88 (76.905, -5.401) -> (76.905, -6.9623)
  arc A43 (75.7758, -8.576) -> (76.905, -6.9623) centre (76.4829, -7.8689) ccw
  line L89 (75.7758, -8.576) -> (68.2242, -8.576)
  arc A44 (67.095, -6.9623) -> (68.2242, -8.576) centre (67.5171, -7.8689) ccw
  line L90 (67.095, -6.9623) -> (67.095, -5.401)
  line L91 (67.095, -5.401) -> (56.905, -5.401)
  line L92 (56.905, -5.401) -> (56.905, -6.9623)
  arc A45 (55.7758, -8.576) -> (56.905, -6.9623) centre (56.4829, -7.8689) ccw
  line L93 (55.7758, -8.576) -> (48.2242, -8.576)
  arc A46 (47.095, -6.9623) -> (48.2242, -8.576) centre (47.5171, -7.8689) ccw
  line L94 (47.095, -6.9623) -> (47.095, -5.401)
  line L95 (47.095, -5.401) -> (36.905, -5.401)
  line L96 (36.905, -5.401) -> (36.905, -6.9623)
  arc A47 (35.7758, -8.576) -> (36.905, -6.9623) centre (36.4829, -7.8689) ccw
  line L97 (35.7758, -8.576) -> (28.2242, -8.576)
  arc A48 (27.095, -6.9623) -> (28.2242, -8.576) centre (27.5171, -7.8689) ccw
  line L98 (27.095, -6.9623) -> (27.095, -5.401)
  line L99 (27.095, -5.401) -> (16.905, -5.401)
  line L100 (16.905, -5.401) -> (16.905, -6.9623)
  arc A49 (15.7758, -8.576) -> (16.905, -6.9623) centre (16.4829, -7.8689) ccw
  line L101 (15.7758, -8.576) -> (5.175, -8.576)
  line L102 (5.175, -8.576) -> (5.175, -10.211)
  arc A50 (5.175, -11.6252) -> (5.175, -10.211) centre (4.4679, -10.9181) ccw
  line L103 (5.175, -11.6252) -> (5.175, -19.1768)
  arc A51 (3.5613, -20.306) -> (5.175, -19.1768) centre (4.4679, -19.8839) ccw
  line L104 (3.5613, -20.306) -> (2, -20.306)
  line L105 (2, -20.306) -> (2, -30.496)
  line L106 (2, -30.496) -> (3.5613, -30.496)
  arc A52 (5.175, -31.6252) -> (3.5613, -30.496) centre (4.4679, -30.9181) ccw
  line L107 (5.175, -31.6252) -> (5.175, -39.1768)
  arc A53 (3.5613, -40.306) -> (5.175, -39.1768) centre (4.4679, -39.8839) ccw
  line L108 (3.5613, -40.306) -> (2, -40.306)
  line L109 (2, -40.306) -> (2, -50.496)
  line L110 (2, -50.496) -> (3.5613, -50.496)
  arc A54 (5.175, -51.6252) -> (3.5613, -50.496) centre (4.4679, -50.9181) ccw
  line L111 (5.175, -51.6252) -> (5.175, -59.1768)
  arc A55 (5.175, -60.591) -> (5.175, -59.1768) centre (4.4679, -59.8839) ccw
sketch "Plaform" plane through (0, 0, 0) normal (0, 0, 1) x (1, 0, 0) in component "Platform"
  line L0 (-255.6038, 317) -> (-88.6038, 317)
  line L1 (-85.6038, 314) -> (-85.6038, 203)
  line L2 (-88.6038, 200) -> (-255.6038, 200)
  line L3 (-258.6038, 203) -> (-258.6038, 314)
  line L4 (1.75, 0) -> (22.5, 0)
  line L5 (0, 1.75) -> (0, 22.5)
  line L6 (-178.6038, 263) -> (-165.6038, 263)
  line L7 (-163.6038, 261) -> (-163.6038, 256)
  line L8 (-165.6038, 254) -> (-178.6038, 254)
  line L9 (-180.6038, 256) -> (-180.6038, 261)
  line L10 (-187.1038, 314) -> (-157.1038, 314) construction
  line L11 (-157.1038, 314) -> (-157.1038, 203) construction
  line L12 (-157.1038, 203) -> (-187.1038, 203) construction
  line L13 (-187.1038, 203) -> (-187.1038, 314) construction
  line L14 (-187.1038, 314) -> (-157.1038, 203) construction
  line L15 (-157.1038, 314) -> (-187.1038, 203) construction
  circle A0 centre (-187.1038, 314) radius 1.5
  circle A1 centre (-157.1038, 314) radius 1.5
  circle A2 centre (-157.1038, 203) radius 1.5
  circle A3 centre (-187.1038, 203) radius 1.5
  line L16 (-239.1038, 305) -> (-105.1038, 305) construction
  line L17 (-105.1038, 212) -> (-239.1038, 212) construction
  line L18 (-239.1038, 212) -> (-239.1038, 305) construction
  line L19 (-239.1038, 305) -> (-105.1038, 212) construction
  line L20 (-105.1038, 305) -> (-239.1038, 212) construction
  line L21 (-89.1038, 203.5) -> (-255.1038, 203.5) construction
  line L22 (-255.1038, 203.5) -> (-255.1038, 313.5) construction
  line L23 (-255.1038, 313.5) -> (-89.1038, 313.5) construction
  line L24 (-89.1038, 203.5) -> (-255.1038, 313.5) construction
  line L25 (-255.1038, 203.5) -> (-89.1038, 313.5) construction
  circle A4 centre (-255.1038, 203.5) radius 1.75
  circle A5 centre (-255.1038, 313.5) radius 1.75
  circle A6 centre (-89.1038, 313.5) radius 1.75
  circle A7 centre (-89.1038, 203.5) radius 1.75
  circle A8 centre (-118.6038, 258.5) radius 1.5
  circle A9 centre (-88.6038, 258.5) radius 1.5
  arc A10 (-88.6038, 200) -> (-85.6038, 203) centre (-88.6038, 203) ccw
  arc A11 (-258.6038, 203) -> (-255.6038, 200) centre (-255.6038, 203) ccw
  arc A12 (-255.6038, 317) -> (-258.6038, 314) centre (-255.6038, 314) ccw
  arc A13 (-85.6038, 314) -> (-88.6038, 317) centre (-88.6038, 314) ccw
  circle A14 centre (-239.1038, 305) radius 1.75
  circle A15 centre (-105.1038, 305) radius 1.75
  circle A16 centre (-105.1038, 212) radius 1.75
  circle A17 centre (-239.1038, 212) radius 1.75
  line L26 (-105.1038, 305) -> (-105.1038, 212) construction
  arc A18 (-178.6038, 263) -> (-180.6038, 261) centre (-178.6038, 261) ccw
  arc A19 (-163.6038, 261) -> (-165.6038, 263) centre (-165.6038, 261) ccw
  arc A20 (-180.6038, 256) -> (-178.6038, 254) centre (-178.6038, 256) ccw
  arc A21 (-165.6038, 254) -> (-163.6038, 256) centre (-165.6038, 256) ccw
  point P0 (-258.6038, 317)
  point P1 (-85.6038, 317)
  point P2 (-258.6038, 200)
  point P3 (-180.6038, 263)
  point P4 (-163.6038, 263)
  point P5 (-180.6038, 254)
  point P6 (-85.6038, 258.5)
  point P7 (-172.1038, 263)
  point P8 (-172.1038, 317)
  point P9 (-172.1038, 258.5)
  point P10 (-172.1038, 258.5)
  point P11 (-172.1038, 258.5)
  point P12 (-258.6038, 258.5)
  point P13 (-172.1038, 200)
  point P14 (-255.1038, 258.5)
  point P15 (-180.6038, 258.5)
  point P16 (-172.1038, 254)
  dimension "d1498" = 173
  dimension "d1499" = 117
  dimension "d1500" = 200
  dimension "d1501" = 85.6038
  dimension "d1502" = 17
  dimension "d1503" = 9
  dimension "d1505" = 30
  dimension "d1506" = 111
  dimension "d1507" = 3
  dimension "d1508" = 3
  dimension "d1509" = 3
  dimension "d1510" = 3
  dimension "d1512" = 93
  dimension "d1513" = 166
  dimension "d1514" = 110
  dimension "d1515" = 3.5
  dimension "d1516" = 3.5
  dimension "d1517" = 3.5
  dimension "d1518" = 3.5
  dimension "d1552" = 3
  dimension "d1553" = 3
  dimension "d1554" = 3
  dimension "d1555" = 3
  dimension "d1557" = 3.5
  dimension "d1558" = 3.5
  dimension "d1559" = 3.5
  dimension "d1560" = 3.5
  dimension "d1611" = 3
  dimension "d1612" = 3
  dimension "d1613" = 3
  dimension "d1614" = 30
  dimension "d1615" = 134
  dimension "d1650" = 2
  dimension "d1651" = 2
  dimension "d1652" = 2
  dimension "d1653" = 2
  dimension "d1736" = 9
  constraint horizontal L0
  constraint vertical L1
  constraint horizontal L2
  constraint vertical L3
  constraint horizontal L6
  constraint vertical L7
  constraint horizontal L8
  constraint vertical L9
  constraint vertical P7 P8
  constraint horizontal L10
  constraint perpendicular L10 L11
  constraint parallel L10 L12
  constraint parallel L11 L13
  constraint coincident L14 P11
  constraint coincident L15 P11
  constraint horizontal P6 P10
  constraint vertical P8 P11
  constraint coincident L10.start L13.end
  constraint coincident L10.end L11.start
  constraint coincident L11.end L12.start
  constraint coincident L12.end L13.start
  constraint horizontal L16
  constraint parallel L16 L17
  constraint coincident L19 P11
  constraint coincident L20 P11
  constraint coincident P11 P10
  constraint horizontal L21
  constraint perpendicular L21 L22
  constraint parallel L21 L23
  constraint coincident L24 P11
  constraint coincident L25 P11
  constraint coincident L21.end L22.start
  constraint coincident L22.end L23.start
  constraint coincident L23.end L25.end
  constraint coincident L21.start L24.start
  constraint coincident L1 P6
  constraint tangent L2 A10
  constraint tangent L1 A10
  constraint coincident P2 L2
  constraint coincident P2 L3
  constraint tangent L2 A11
  constraint tangent L3 A11
  constraint coincident L0 P8
  constraint coincident P0 L3
  constraint coincident P0 L0
  constraint tangent L3 A12
  constraint tangent L0 A12
  constraint midpoint L3 P12
  constraint horizontal P11 P12
  constraint midpoint L2 P13
  constraint vertical P11 P13
  constraint coincident P1 L0
  constraint coincident P1 L1
  constraint tangent L0 A13
  constraint tangent L1 A13
  constraint coincident L16.start L18.end
  constraint coincident L16.end L20.start
  constraint coincident L17.start L19.end
  constraint coincident L17.end L18.start
  constraint perpendicular L17 L26
  constraint perpendicular L17 L18
  constraint horizontal A8.centre A9.centre
  constraint horizontal P6 A9.centre
  constraint midpoint L22 P14
  constraint horizontal P12 P14
  constraint coincident L6 P7
  constraint coincident P3 L9
  constraint coincident P3 L6
  constraint tangent L9 A18
  constraint tangent L6 A18
  constraint coincident P4 L6
  constraint coincident P4 L7
  constraint tangent L6 A19
  constraint tangent L7 A19
  constraint coincident P5 L9
  constraint coincident P5 L8
  constraint tangent L9 A20
  constraint tangent L8 A20
  constraint tangent L8 A21
  constraint tangent L7 A21
  constraint midpoint L9 P15
  constraint horizontal P11 P15
  constraint midpoint L8 P16
  constraint vertical P11 P16
  measures "d1498" distance of P0 P1
  measures "d1499" distance of P0 P2
  measures "d1500" distance of L2 L4
  measures "d1501" distance of L1 L5
  measures "d1502" distance of P3 P4
  measures "d1503" distance of P3 P5
  measures "d1505" distance of L11.end L12.end
  measures "d1506" distance of L10.start L12.end
  measures "d1507" diameter of A0
  measures "d1508" diameter of A1
  measures "d1509" diameter of A2
  measures "d1510" diameter of A3
  measures "d1512" distance of L16 L17
  measures "d1513" distance of L22.end L23.end
  measures "d1514" distance of L21.end L22.end
  measures "d1515" diameter of A4
  measures "d1516" diameter of A5
  measures "d1517" diameter of A6
  measures "d1518" diameter of A7
  measures "d1552" radius of A10
  measures "d1553" radius of A11
  measures "d1554" radius of A12
  measures "d1555" radius of A13
  measures "d1557" diameter of A14
  measures "d1558" diameter of A15
  measures "d1559" diameter of A16
  measures "d1560" diameter of A17
  measures "d1611" distance of L1 A9.centre
  measures "d1612" diameter of A8
  measures "d1613" diameter of A9
  measures "d1614" distance of A8.centre A9.centre
  measures "d1615" distance of L17.start L17.end
  measures "d1650" radius of A18
  measures "d1651" radius of A19
  measures "d1652" radius of A20
  measures "d1653" radius of A21
  measures "d1736" distance of L6 L8
extrude "Extrude1" [suppressed] in component "Platform"
copy_body "CopyPasteBodies12" [suppressed]
move_body "Move37" [suppressed]
copy_body "Body->Comp12" [suppressed] in component "Brace"